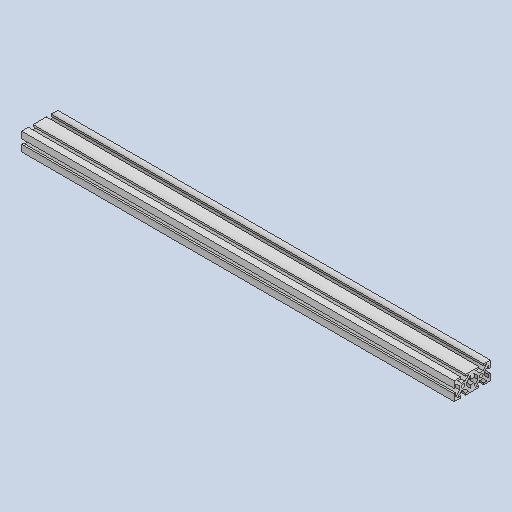
# Autodesk Inventor part: LatX24in1
Saved by Autodesk Inventor 2023 (Build 270158030, 158C)
## iProperties
Created: 2022-06-29
Part Number: LatX24in1
Material: Generic
Document SubType Name: Modeling
Designer: jeremyy
Density: 1 g/cm^3
Appearance: Default
Author: jeremyy
Autodesk Inventor part; units mm, degrees
ref_plane "YZ Plane" through (0, 0, 0) normal (1, 0, 0) x (0, 1, 0)
ref_plane "XZ Plane" through (0, 0, 0) normal (0, 1, 0) x (-1, 0, 0)
ref_plane "XY Plane" through (0, 0, 0) normal (0, 0, 1) x (1, 0, 0)
sketch "Sketch1" plane through (0, 0, 0) normal (1, 0, 0) x (0, 1, 0)
  line L0 (0, 0) -> (0, -9.398)
  line L1 (0, -9.398) -> (2.4765, -9.398)
  line L2 (9.398, -2.4765) -> (9.398, 0)
  line L3 (9.398, 0) -> (0, 0)
  line L4 (16.002, 0) -> (16.002, -2.4765)
  line L5 (22.9235, -9.398) -> (25.4, -9.398)
  line L6 (25.4, -9.398) -> (25.4, 0)
  line L7 (25.4, 0) -> (16.002, 0)
  line L8 (25.4, -16.002) -> (22.9235, -16.002)
  line L9 (16.002, -22.9235) -> (16.002, -25.4)
  line L10 (25.4, -25.4) -> (25.4, -16.002)
  line L11 (0, -16.002) -> (2.4765, -16.002)
  line L12 (9.398, -22.9235) -> (9.398, -25.4)
  line L13 (0, -25.4) -> (0, -16.002)
  line L14 (22.9235, -9.398) -> (22.9235, -4.953)
  line L15 (16.002, -2.4765) -> (20.447, -2.4765)
  line L16 (20.447, -2.4765) -> (15.0495, -7.874)
  line L17 (20.447, -2.4765) -> (28.0802, -2.4765) construction
  line L18 (22.9235, -4.953) -> (17.526, -10.3505)
  line L19 (22.9235, -16.002) -> (22.9235, -20.447)
  line L20 (22.9235, -20.447) -> (17.526, -15.0495)
  line L21 (16.002, -22.9235) -> (20.447, -22.9235)
  line L22 (20.447, -22.9235) -> (15.0495, -17.526)
  line L23 (2.4765, -16.002) -> (2.4765, -20.447)
  line L24 (2.4765, -20.447) -> (7.874, -15.0495)
  line L25 (9.398, -22.9235) -> (4.953, -22.9235)
  line L26 (4.953, -22.9235) -> (10.3505, -17.526)
  line L27 (9.398, -2.4765) -> (4.953, -2.4765)
  line L28 (4.953, -2.4765) -> (10.3505, -7.874)
  line L29 (2.4765, -9.398) -> (2.4765, -4.953)
  line L30 (2.4765, -4.953) -> (7.874, -10.3505)
  line L31 (10.3505, -7.874) -> (15.0495, -7.874)
  line L32 (17.526, -10.3505) -> (17.526, -15.0495)
  line L33 (10.3505, -17.526) -> (15.0495, -17.526)
  line L34 (7.874, -15.0495) -> (7.874, -10.3505)
  circle A0 centre (12.7, -12.7) radius 2.54
  line L35 (0, -50.8) -> (0, -41.402)
  line L36 (0, -41.402) -> (2.4765, -41.402)
  line L37 (9.398, -48.3235) -> (9.398, -50.8)
  line L38 (9.398, -50.8) -> (0, -50.8)
  line L39 (16.002, -50.8) -> (16.002, -48.3235)
  line L40 (22.9235, -41.402) -> (25.4, -41.402)
  line L41 (25.4, -41.402) -> (25.4, -50.8)
  line L42 (25.4, -50.8) -> (16.002, -50.8)
  line L43 (25.4, -34.798) -> (22.9235, -34.798)
  line L44 (16.002, -27.8765) -> (16.002, -25.4)
  line L45 (25.4, -25.4) -> (25.4, -34.798)
  line L46 (0, -34.798) -> (2.4765, -34.798)
  line L47 (9.398, -27.8765) -> (9.398, -25.4)
  line L48 (0, -25.4) -> (0, -34.798)
  line L49 (22.9235, -41.402) -> (22.9235, -45.847)
  line L50 (16.002, -48.3235) -> (20.447, -48.3235)
  line L51 (20.447, -48.3235) -> (15.0495, -42.926)
  line L52 (20.447, -48.3235) -> (28.0802, -48.3235) construction
  line L53 (22.9235, -45.847) -> (17.526, -40.4495)
  line L54 (22.9235, -34.798) -> (22.9235, -30.353)
  line L55 (22.9235, -30.353) -> (17.526, -35.7505)
  line L56 (16.002, -27.8765) -> (20.447, -27.8765)
  line L57 (20.447, -27.8765) -> (15.0495, -33.274)
  line L58 (2.4765, -34.798) -> (2.4765, -30.353)
  line L59 (2.4765, -30.353) -> (7.874, -35.7505)
  line L60 (9.398, -27.8765) -> (4.953, -27.8765)
  line L61 (4.953, -27.8765) -> (10.3505, -33.274)
  line L62 (9.398, -48.3235) -> (4.953, -48.3235)
  line L63 (4.953, -48.3235) -> (10.3505, -42.926)
  line L64 (2.4765, -41.402) -> (2.4765, -45.847)
  line L65 (2.4765, -45.847) -> (7.874, -40.4495)
  line L66 (10.3505, -42.926) -> (15.0495, -42.926)
  line L67 (17.526, -40.4495) -> (17.526, -35.7505)
  line L68 (10.3505, -33.274) -> (15.0495, -33.274)
  line L69 (7.874, -35.7505) -> (7.874, -40.4495)
  circle A1 centre (12.7, -38.1) radius 2.54
  dimension "d2" = 9.398
  dimension "d3" = 2.4765
  dimension "d7" = 2.4765
  dimension "d10" = 2.4765
  dimension "d11" = 25.4
  dimension "d13" = 2.4765
  dimension "d16" = 2.4765
  dimension "d17" = 9.398
  dimension "d23" = 2.4765
  dimension "d25" = 25.4
  dimension "d32" = 4.445
  dimension "d33" = 4.445
  dimension "d35" = 135
  dimension "d36" = 4.445
  dimension "d37" = 4.445
  dimension "d38" = 2.4765
  dimension "d40" = 4.445
  dimension "d41" = 4.445
  dimension "d42" = 4.445
  dimension "d43" = 4.445
  dimension "d44" = 5.08
  constraints: 140 end point, 10 perpendicular, 4 horizontal, 4 vertical, 3 parallel, 2 centre point, 1 equal length
  measures "d2" distance of L0.start L0.end
  measures "d3" distance of L0.end L1.end
  measures "d7" distance of L4.start L4.end
  measures "d10" distance of L5.start L5.end
  measures "d11" distance between parallel lines of L0 L6
  measures "d13" distance of L8.start L8.end
  measures "d16" distance of L9.start L9.end
  measures "d17" distance of L9.end L10.start
  measures "d23" distance of L12.start L12.end
  measures "d25" distance between parallel lines of L10 L13
  measures "d32" distance of L5.start L14.end
  measures "d33" distance of L4.end L15.end
  measures "d35" angle of L16 L17
  measures "d36" distance of L8.end L19.end
  measures "d37" distance of L9.start L21.end
  measures "d38" distance of L2.start L2.end
  measures "d40" distance of L11.end L23.end
  measures "d41" distance of L12.start L25.end
  measures "d42" distance of L2.start L27.end
  measures "d43" distance of L1.end L29.end
  measures "d44" diameter of A0
extrude "Extrusion1" add sketch "Sketch1" along normal blind 609.6
body "Solid1"
